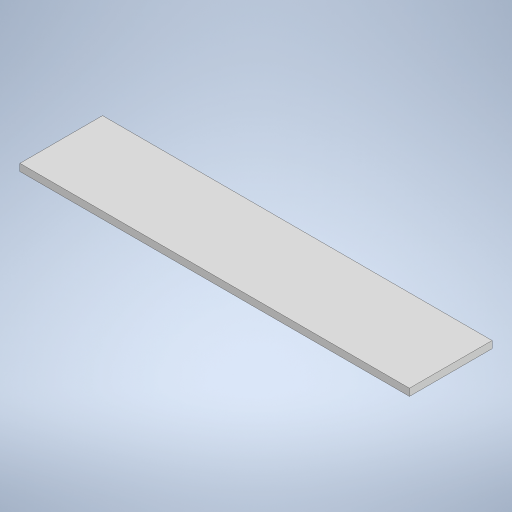
# Autodesk Inventor part: Brazo mdf 2
Saved by Autodesk Inventor 2023 (Build 270158000, 158)
## iProperties
Created: 2022-11-02
Part Number: Brazo mdf 2
Material: Generic
Document SubType Name: Modeling
Designer: diego
Density: 1 g/cm^3
Appearance: Default
Author: diego
Autodesk Inventor part; units mm, degrees
ref_plane "YZ Plane" through (0, 0, 0) normal (1, 0, 0) x (0, 1, 0)
ref_plane "XZ Plane" through (0, 0, 0) normal (0, 1, 0) x (-1, 0, 0)
ref_plane "XY Plane" through (0, 0, 0) normal (0, 0, 1) x (1, 0, 0)
sketch "Sketch1" plane through (0, 0, 0) normal (0, 1, 0) x (-1, 0, 0)
  line L0 (0, 0) -> (0, -35)
  line L1 (0, -35) -> (-165, -35)
  line L2 (-165, -35) -> (-165, 0)
  line L3 (-165, 0) -> (0, 0)
  dimension "d0" = 35
  dimension "d1" = 165
  constraints: 8 end point, 3 perpendicular, 1 vertical
  measures "d0" distance of L0.start L0.end
  measures "d1" distance of L0.end L1.end
extrude "Extrusion1" add sketch "Sketch1" along normal blind 3
body "Solid1"
